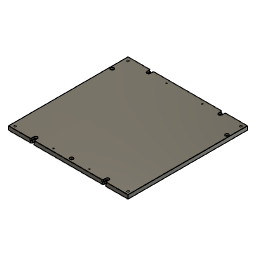
Voron Plate 250x250 Universal v2 (Autodesk Fusion 360 design; units mm, degrees)
Autodesk Fusion 360 part; units mm, degrees
note: some values were not read from the file. Chosen so that the rebuilt part matches the saved one: which face or edge a step refers to; how an offset face is resized; which pieces of a blend or face edit are solid.
sketch "Sketch1" plane through (0, 0, 0) normal (0, 1, 0) x (1, 0, 0)
  line L0 (0, 0) -> (250, 0)
  line L1 (250, 0) -> (250, 250)
  line L2 (250, 250) -> (0, 250)
  line L3 (0, 250) -> (0, 0)
  line L4 (125, 0) -> (50, 0) construction
  line L5 (50, 0) -> (50, 7) construction
  line L6 (50, 7) -> (200, 7) construction
  line L7 (125, 250) -> (125, 243) construction
  line L8 (125, 243) -> (50, 243) construction
  line L9 (50, 243) -> (200, 243) construction
  circle A0 centre (50, 243) radius 1.7
  circle A1 centre (50, 243) radius 3.25
  circle A2 centre (200, 243) radius 1.7
  circle A3 centre (200, 243) radius 3.25
  circle A4 centre (50, 7) radius 1.7
  circle A5 centre (50, 7) radius 3.25
  circle A6 centre (200, 7) radius 1.7
  circle A7 centre (200, 7) radius 3.25
  line L10 (0, 0) -> (7, 0)
  line L11 (7, 0) -> (7, 7) construction
  line L12 (7, 7) -> (0, 7) construction
  line L13 (0, 7) -> (0, 0)
  circle A8 centre (7, 7) radius 2.1
  line L14 (250, 0) -> (243, 0)
  line L15 (243, 0) -> (243, 7) construction
  line L16 (243, 7) -> (250, 7) construction
  line L17 (250, 7) -> (250, 0)
  circle A9 centre (243, 7) radius 2.1
  dimension "d1" = 250
  dimension "d2" = 250
  dimension "d3" = 75
  dimension "d4" = 7
  dimension "d5" = 150
  dimension "d6" = 7
  dimension "d7" = 75
  dimension "d8" = 150
  dimension "d9" = 3.4
  dimension "d10" = 6.5
  dimension "d11" = 3.4
  dimension "d12" = 6.5
  dimension "d13" = 3.4
  dimension "d14" = 6.5
  dimension "d15" = 3.4
  dimension "d16" = 6.5
  dimension "d17" = 7
  dimension "d18" = 7
  dimension "d19" = 4.2
  dimension "d20" = 7
  dimension "d21" = 7
  dimension "d22" = 4.2
  constraint horizontal L0
  constraint vertical L1
  constraint horizontal L2
  constraint vertical L3
  constraint coincident L0.start L3.end
  constraint midpoint L0 L4.start
  constraint perpendicular L3 L4
  constraint vertical L5
  constraint perpendicular L5 L6
  constraint midpoint L2 L7.start
  constraint vertical L7
  constraint perpendicular L7 L8
  constraint parallel L8 L9
  constraint coincident L8.end L9.start
  constraint concentric A0 A1
  constraint coincident L9.end A2.centre
  constraint concentric A2 A3
  constraint coincident L5.end L6.start
  constraint concentric A4 A5
  constraint coincident L6.end A6.centre
  constraint concentric A6 A7
  constraint horizontal L10
  constraint vertical L11
  constraint horizontal L12
  constraint vertical L13
  constraint coincident L11.end L12.start
  constraint horizontal L14
  constraint vertical L15
  constraint horizontal L16
  constraint vertical L17
  constraint coincident L15.end L16.start
  measures "d1" distance of L0.start L0.end
  measures "d2" distance of L0.start L2.end
  measures "d3" distance of L4.start L4.end
  measures "d4" distance of L4.end L5.end
  measures "d5" distance of L5.end L6.end
  measures "d6" distance of L7.start L7.end
  measures "d7" distance of L7.end L8.end
  measures "d8" distance of L8.end L9.end
  measures "d9" diameter of A0
  measures "d10" diameter of A1
  measures "d11" diameter of A2
  measures "d12" diameter of A3
  measures "d13" diameter of A4
  measures "d14" diameter of A5
  measures "d15" diameter of A6
  measures "d16" diameter of A7
  measures "d17" distance of L0.start L10.end
  measures "d18" distance of L0.start L12.end
  measures "d19" diameter of A8
  measures "d20" distance of L0.end L14.end
  measures "d21" distance of L0.end L16.end
  measures "d22" diameter of A9
extrude "Extrude1" add sketch "Sketch1" along normal blind 8 contours L0 L1 L2 L3 L10 L13 L14 L17 | A1 | A3 | A5 | A7 | A8 | A9
extrude "Extrude2" cut sketch "Sketch1" along normal blind 30 and the other way blind -4.5 contours A1 | A3 | A5 | A7
extrude "Extrude3" cut sketch "Sketch1" along normal blind 6 contours A8 | A9
thread "Thread1" "ISO Metric profile 5.0 M5x0.8 6H" major diameter 5.12 minor diameter 4.234 pitch 0.8 angle 60 resizes the face on face at (243.0524, 4, -9.0993) on face at (9.0974, 4, -6.8953)
fillet "Fillet2" radius 0.2 4 edges at (250, 4, 0) (250, 4, -250) (0, 4, 0) (0, 4, -250)
sketch "Sketch2" plane through (0, 8, 0) normal (0, 1, 0) x (-1, 0, 0)
  arc A0 (-0.2, -250) -> (0, -249.8) centre (-0.2, -249.8) ccw
  line L0 (0, -249.8) -> (0, -0.2)
  arc A1 (0, -0.2) -> (-0.2, 0) centre (-0.2, -0.2) ccw
  line L1 (-0.2, 0) -> (-249.8, 0)
  arc A2 (-249.8, 0) -> (-250, -0.2) centre (-249.8, -0.2) ccw
  line L2 (-250, -0.2) -> (-250, -249.8)
  arc A3 (-250, -249.8) -> (-249.8, -250) centre (-249.8, -249.8) ccw
  line L3 (-249.8, -250) -> (-0.2, -250)
  circle A4 centre (-200, -243) radius 3.25
  circle A5 centre (-200, -7) radius 3.25
  circle A6 centre (-50, -243) radius 3.25
  circle A7 centre (-50, -7) radius 3.25
  line L4 (-200, -7) -> (-203.25, -7) construction
  line L5 (-200, -7) -> (-200, 0) construction
  line L6 (-203.25, -7) -> (-203.25, 0)
  line L7 (-196.75, -7) -> (-196.75, 0)
  constraint coincident A5.centre L4.start
  constraint coincident A5 L4.end
  constraint parallel L1 L4
  constraint coincident L1 L5.end
  constraint perpendicular L1 L5
  constraint coincident L1 L6.end
  constraint tangent A5 L6
  constraint symmetric L4.end L5 L7.start
  constraint symmetric L5 L6.end L7.end
extrude "Extrude4" cut sketch "Sketch2" against normal blind 3.5 contours L1 A5 L6 L7
sketch "Sketch3" plane through (0, 4.5, 0) normal (0, 1, 0) x (-1, 0, 0)
  circle A0 centre (-200, -7) radius 1.7
  arc A1 (-203.25, -7) -> (-196.75, -7) centre (-200, -7) ccw
  line L0 (-196.75, -7) -> (-196.75, 0)
  line L1 (-196.75, 0) -> (-203.25, 0)
  line L2 (-203.25, 0) -> (-203.25, -7)
  line L3 (-200, -7) -> (-201.7, -7) construction
  line L4 (-201.7, -7) -> (-201.7, 0)
  line L5 (-200, -7) -> (-198.3, -7) construction
  line L6 (-198.3, -7) -> (-198.3, 0)
  constraint coincident A0.centre A1.centre
  constraint coincident A0 L3.end
  constraint parallel L1 L3
  constraint coincident L1 L4.end
  constraint tangent A0 L4
  constraint coincident A0 L5.end
  constraint parallel L3 L5
  constraint coincident L1 L6.end
  constraint tangent A0 L6
extrude "Extrude5" cut sketch "Sketch3" against normal blind 11 contours A0 L1 L4 L6
fillet "Fillet3" radius 2 4 edges at (203.25, 6.25, 0) (196.75, 6.25, 0) (201.7, 2.25, 0) (198.3, 2.25, 0)
ref_plane "WorkPlane1" through (125, 4, -125) normal (-1, 0, 0) x (0, 0, 1)
mirror "Mirror1" about plane through (125, 4, -125) normal (-1, 0, 0) of 11 faces at (195.1285, 6.8333, -0.0361) (204.7785, 6.8333, -0.0564) (203.25, 5.6667, -5.3333) (202.7333, 4.5, -3.6667) (198.3084, 1.5, -7.1693) (203.2339, 6.8333, -7.3236) (196.75, 6.8333, -5.3333) (195.1285, 6.8333, -0.0361) (196.6785, 3, -0.0361) (198.3, 3, -5.3333) (201.7, 3, -5.3333)
ref_plane "WorkPlane3" through (23.25, 4, -125) normal (0, 0, 1) x (1, 0, 0)
mirror "Mirror2" about plane through (23.25, 4, -125) normal (0, 0, 1) of 22 faces at (204.7785, 6.8333, -0.0564) (46.7477, 6.8333, -1.9048) (52.7333, 4.5, -3.6667) (53.246, 5.6667, -7.162) (195.1285, 6.8333, -0.0361) (51.6979, 1.5, -7.0847) (198.3, 3, -5.3333) (196.75, 6.8333, -5.3333) (55.1548, 6.8333, -0.0023) (203.25, 5.6667, -5.3333) (201.7, 3, -5.3333) (196.6785, 3, -0.0361) (48.3, 3, -5.3333) (198.3084, 1.5, -7.1693) (53.5099, 1.5, -0.0091) (195.1285, 6.8333, -0.0361) (202.7333, 4.5, -3.6667) (53.25, 5.6667, -5.3333) (203.2339, 6.8333, -7.3236) (51.7, 3, -5.3333) (204.7785, 6.8333, -0.0564) (46.75, 5.6667, -5.3333)
chamfer "Chamfer4" distance 0.2 angle 45 32 edges at (203.8358, 8, -249.4142) (203.25, 8, -245.5) (200, 8, -239.75) (196.75, 8, -245.5) (196.1642, 8, -249.4142) (125, 8, -250) (53.8358, 8, -249.4142) (53.25, 8, -245.5) (50, 8, -239.75) (46.75, 8, -245.5) (46.1642, 8, -249.4142) (22.475, 8, -250) (0.0586, 8, -249.9414) (0, 8, -125) (0.0586, 8, -0.0586) (22.475, 8, 0) (46.1642, 8, -0.5858) (46.75, 8, -4.5) (50, 8, -10.25) (53.25, 8, -4.5) (53.8358, 8, -0.5858) (125, 8, 0) (196.1642, 8, -0.5858) (196.75, 8, -4.5) (200, 8, -10.25) (203.25, 8, -4.5) (203.8358, 8, -0.5858) (227.525, 8, 0) (249.9414, 8, -0.0586) (250, 8, -125) (249.9414, 8, -249.9414) (227.525, 8, -250)
delete_face "DeleteFace1" 1 faces at (9.1144, 2, -7.1055)
delete_face "DeleteFace2" 1 faces at (242.0342, 2, -5.1161)
chamfer "Chamfer5" distance 0.2 angle 45 32 edges at (23.25, 0, 0) (47.7142, 0, -0.5858) (48.3, 0, -4.5) (50, 0, -8.7) (51.7, 0, -4.5) (52.2858, 0, -0.5858) (125, 0, 0) (197.7142, 0, -0.5858) (198.3, 0, -4.5) (200, 0, -8.7) (201.7, 0, -4.5) (202.2858, 0, -0.5858) (226.75, 0, 0) (249.9414, 0, -0.0586) (250, 0, -125) (249.9414, 0, -249.9414) (226.75, 0, -250) (202.2858, 0, -249.4142) (201.7, 0, -245.5) (200, 0, -241.3) (198.3, 0, -245.5) (197.7142, 0, -249.4142) (125, 0, -250) (52.2858, 0, -249.4142) (51.7, 0, -245.5) (50, 0, -241.3) (48.3, 0, -245.5) (47.7142, 0, -249.4142) (23.25, 0, -250) (0.0586, 0, -249.9414) (0, 0, -125) (0.0586, 0, -0.0586)
sketch "Sketch4" plane through (0, 8, 0) normal (0, 1, 0) x (-1, 0, 0)
  arc A0 (-205.25, -249.8) -> (-203.45, -248) centre (-205.25, -248) ccw
  line L0 (-203.45, -248) -> (-203.45, -243)
  arc A1 (-196.55, -243) -> (-203.45, -243) centre (-200, -243) ccw
  line L1 (-196.55, -243) -> (-196.55, -248)
  arc A2 (-196.55, -248) -> (-194.75, -249.8) centre (-194.75, -248) ccw
  line L2 (-194.75, -249.8) -> (-55.25, -249.8)
  arc A3 (-55.25, -249.8) -> (-53.45, -248) centre (-55.25, -248) ccw
  line L3 (-53.45, -248) -> (-53.45, -243)
  arc A4 (-46.55, -243) -> (-53.45, -243) centre (-50, -243) ccw
  line L4 (-46.55, -243) -> (-46.55, -248)
  arc A5 (-46.55, -248) -> (-44.75, -249.8) centre (-44.75, -248) ccw
  line L5 (-44.75, -249.8) -> (-0.2, -249.8)
  line L6 (-0.2, -249.8) -> (-0.2, -0.2)
  line L7 (-0.2, -0.2) -> (-44.75, -0.2)
  arc A6 (-44.75, -0.2) -> (-46.55, -2) centre (-44.75, -2) ccw
  line L8 (-46.55, -2) -> (-46.55, -7)
  arc A7 (-53.45, -7) -> (-46.55, -7) centre (-50, -7) ccw
  line L9 (-53.45, -7) -> (-53.45, -2)
  arc A8 (-53.45, -2) -> (-55.25, -0.2) centre (-55.25, -2) ccw
  line L10 (-55.25, -0.2) -> (-194.75, -0.2)
  arc A9 (-194.75, -0.2) -> (-196.55, -2) centre (-194.75, -2) ccw
  line L11 (-196.55, -2) -> (-196.55, -7)
  arc A10 (-203.45, -7) -> (-196.55, -7) centre (-200, -7) ccw
  line L12 (-203.45, -7) -> (-203.45, -2)
  arc A11 (-203.45, -2) -> (-205.25, -0.2) centre (-205.25, -2) ccw
  line L13 (-205.25, -0.2) -> (-249.8, -0.2)
  line L14 (-249.8, -0.2) -> (-249.8, -249.8)
  line L15 (-249.8, -249.8) -> (-205.25, -249.8)
  line L16 (-55.25, 0) -> (-194.75, 0)
  line L17 (-125, 0) -> (-125, -7) construction
  circle A12 centre (-125, -7) radius 1.7
  circle A13 centre (-125, -7) radius 3.25
  line L18 (-194.75, -250) -> (-55.25, -250)
  line L19 (-125, -250) -> (-125, -212) construction
  line L20 (-125, -212) -> (-245, -212) construction
  circle A14 centre (-245, -212) radius 1.7
  circle A15 centre (-245, -212) radius 3.25
  circle A16 centre (-5, -212) radius 3.25
  circle A17 centre (-5, -212) radius 1.7
  dimension "d48" = 7
  dimension "d49" = 3.4
  dimension "d50" = 6.5
  dimension "d51" = 38
  dimension "d52" = 120
  dimension "d53" = 3.4
  dimension "d54" = 6.5
  constraint midpoint L16 L17.start
  constraint perpendicular L10 L17
  constraint coincident L17.end A12.centre
  constraint concentric A12 A13
  constraint midpoint L18 L19.start
  constraint perpendicular L2 L19
  constraint perpendicular L19 L20
  constraint coincident L20.end A14.centre
  constraint concentric A14 A15
  constraint symmetric L19 A14 A17
  constraint symmetric L19 A15 A16
  measures "d48" distance of L17.start L17.end
  measures "d49" diameter of A12
  measures "d50" diameter of A13
  measures "d51" distance of L19.start L19.end
  measures "d52" distance of L19.end L20.end
  measures "d53" diameter of A14
  measures "d54" diameter of A15
extrude "Extrude6" cut sketch "Sketch4" against normal blind 40 contours A12 | A14 | A17
extrude "Extrude7" cut sketch "Sketch4" against normal blind 3.5 contours A13 | A15 | A16
chamfer "Chamfer6" distance 0.2 angle 45 3 edges at (8.0301, 8, -210.8247) (128.0301, 8, -5.8247) (248.0301, 8, -210.8247)
sketch "Sketch5" plane through (0, 0, 0) normal (0, -1, 0) x (1, 0, 0)
  circle A0 centre (125, -7) radius 1.7
  circle A1 centre (5, -212) radius 1.7
  circle A2 centre (245, -212) radius 1.7
  line L0 (0.2, -249.8) -> (46.3, -249.8)
  arc A3 (46.3, -249.8) -> (48.1, -248) centre (46.3, -248) ccw
  line L1 (48.1, -248) -> (48.1, -243)
  arc A4 (51.9, -243) -> (48.1, -243) centre (50, -243) ccw
  line L2 (51.9, -243) -> (51.9, -248)
  arc A5 (51.9, -248) -> (53.7, -249.8) centre (53.7, -248) ccw
  line L3 (53.7, -249.8) -> (196.3, -249.8)
  arc A6 (196.3, -249.8) -> (198.1, -248) centre (196.3, -248) ccw
  line L4 (198.1, -248) -> (198.1, -243)
  arc A7 (201.9, -243) -> (198.1, -243) centre (200, -243) ccw
  line L5 (201.9, -243) -> (201.9, -248)
  arc A8 (201.9, -248) -> (203.7, -249.8) centre (203.7, -248) ccw
  line L6 (203.7, -249.8) -> (249.8, -249.8)
  line L7 (249.8, -249.8) -> (249.8, -0.2)
  line L8 (249.8, -0.2) -> (203.7, -0.2)
  arc A9 (203.7, -0.2) -> (201.9, -2) centre (203.7, -2) ccw
  line L9 (201.9, -2) -> (201.9, -7)
  arc A10 (198.1, -7) -> (201.9, -7) centre (200, -7) ccw
  line L10 (198.1, -7) -> (198.1, -2)
  arc A11 (198.1, -2) -> (196.3, -0.2) centre (196.3, -2) ccw
  line L11 (196.3, -0.2) -> (53.7, -0.2)
  arc A12 (53.7, -0.2) -> (51.9, -2) centre (53.7, -2) ccw
  line L12 (51.9, -2) -> (51.9, -7)
  arc A13 (48.1, -7) -> (51.9, -7) centre (50, -7) ccw
  line L13 (48.1, -7) -> (48.1, -2)
  arc A14 (48.1, -2) -> (46.3, -0.2) centre (46.3, -2) ccw
  line L14 (46.3, -0.2) -> (0.2, -0.2)
  line L15 (0.2, -0.2) -> (0.2, -249.8)
  line L16 (0, -250) -> (7, -250) construction
  line L17 (7, -250) -> (7, -243) construction
  line L18 (250, -250) -> (243, -250) construction
  line L19 (243, -250) -> (243, -243) construction
  circle A15 centre (243, -243) radius 2.1
  circle A16 centre (7, -243) radius 2.1
  dimension "d60" = 7
  dimension "d61" = 7
  dimension "d62" = 7
  dimension "d63" = 7
  dimension "d64" = 4.2
  dimension "d65" = 4.2
  constraint horizontal L16
  constraint perpendicular L0 L17
  constraint horizontal L18
  constraint perpendicular L6 L19
  constraint coincident L19.end A15.centre
  constraint coincident L17.end A16.centre
  measures "d60" distance of L16.start L16.end
  measures "d61" distance of L16.end L17.end
  measures "d62" distance of L18.start L18.end
  measures "d63" distance of L18.end L19.end
  measures "d64" diameter of A15
  measures "d65" diameter of A16
extrude "Extrude8" cut sketch "Sketch5" against normal blind 7 contours A15 | A16
sketch "Sketch6" plane through (0, 0, 0) normal (0, -1, 0) x (1, 0, 0)
  circle A0 centre (7, -243) radius 2.1
  circle A1 centre (243, -243) radius 2.1
  circle A2 centre (125, -7) radius 1.7
  circle A3 centre (5, -212) radius 1.7
  circle A4 centre (245, -212) radius 1.7
  line L0 (0.2, -249.8) -> (46.3, -249.8)
  arc A5 (46.3, -249.8) -> (48.1, -248) centre (46.3, -248) ccw
  line L1 (48.1, -248) -> (48.1, -243)
  arc A6 (51.9, -243) -> (48.1, -243) centre (50, -243) ccw
  line L2 (51.9, -243) -> (51.9, -248)
  arc A7 (51.9, -248) -> (53.7, -249.8) centre (53.7, -248) ccw
  line L3 (53.7, -249.8) -> (196.3, -249.8)
  arc A8 (196.3, -249.8) -> (198.1, -248) centre (196.3, -248) ccw
  line L4 (198.1, -248) -> (198.1, -243)
  arc A9 (201.9, -243) -> (198.1, -243) centre (200, -243) ccw
  line L5 (201.9, -243) -> (201.9, -248)
  arc A10 (201.9, -248) -> (203.7, -249.8) centre (203.7, -248) ccw
  line L6 (203.7, -249.8) -> (249.8, -249.8)
  line L7 (249.8, -249.8) -> (249.8, -0.2)
  line L8 (249.8, -0.2) -> (203.7, -0.2)
  arc A11 (203.7, -0.2) -> (201.9, -2) centre (203.7, -2) ccw
  line L9 (201.9, -2) -> (201.9, -7)
  arc A12 (198.1, -7) -> (201.9, -7) centre (200, -7) ccw
  line L10 (198.1, -7) -> (198.1, -2)
  arc A13 (198.1, -2) -> (196.3, -0.2) centre (196.3, -2) ccw
  line L11 (196.3, -0.2) -> (53.7, -0.2)
  arc A14 (53.7, -0.2) -> (51.9, -2) centre (53.7, -2) ccw
  line L12 (51.9, -2) -> (51.9, -7)
  arc A15 (48.1, -7) -> (51.9, -7) centre (50, -7) ccw
  line L13 (48.1, -7) -> (48.1, -2)
  arc A16 (48.1, -2) -> (46.3, -0.2) centre (46.3, -2) ccw
  line L14 (46.3, -0.2) -> (0.2, -0.2)
  line L15 (0.2, -0.2) -> (0.2, -249.8)
  line L16 (53.7, -250) -> (196.3, -250)
  line L17 (196.3, 0) -> (53.7, 0)
  line L18 (125, -250) -> (125, 0) construction
  line L19 (125, -125) -> (204.8645, -125) construction
  line L20 (125, -250) -> (125, -243) construction
  line L21 (125, -243) -> (87.5, -243) construction
  circle A17 centre (87.5, -243) radius 1.25
  circle A18 centre (162.5, -243) radius 1.25
  circle A19 centre (7, -7) radius 2.1
  circle A20 centre (87.5, -7) radius 1.25
  circle A21 centre (162.5, -7) radius 1.25
  circle A22 centre (243, -7) radius 2.1
  dimension "d68" = 7
  dimension "d69" = 37.5
  dimension "d70" = 2.5
  constraint midpoint L16 L18.start
  constraint midpoint L17 L18.end
  constraint midpoint L18 L19.start
  constraint perpendicular L18 L19
  constraint perpendicular L3 L20
  constraint perpendicular L20 L21
  constraint coincident L21.end A17.centre
  constraint symmetric L18 A17 A18
  constraint symmetric A0 L19 A19
  constraint symmetric A1 L19 A22
  constraint symmetric L19 A17 A20
  constraint symmetric L19 A18 A21
  measures "d68" distance of L18.start L20.end
  measures "d69" distance of L20.end L21.end
  measures "d70" diameter of A17
extrude "Extrude9" cut sketch "Sketch6" against normal blind 7 contours A17 | A18 | A19 | A20 | A21 | A22
chamfer "Chamfer2" [suppressed]
chamfer "Chamfer3" [suppressed]
chamfer "Chamfer1" [suppressed]
fillet "Fillet1" [suppressed]
copy_body "Body->Comp1" [suppressed] in component "Component"
equation "d5 = ( 75 * 2 ) * 1 mm"
equation "d8 = ( 75 * 2 ) * 1 mm"
equation "d27 = -8.00 mm + 3.5 mm"
equation "d69 = ( 75 / 2 ) * 1 mm"
